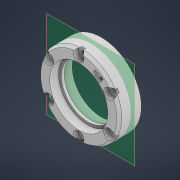
# Autodesk Inventor part: Ring Cover Top
Saved by Autodesk Inventor 2021 (Build 250183000, 183)
## iProperties
Created: 2025-03-19
Part Number: Ring Cover Top
Material: Generic
Document SubType Name: Modeling
Designer: rocke
Density: 0.528258 g/cm^3
Appearance: Default
Mass: 26.1 g
Surface Area: 167.965 cm^2
Volume: 49.4077 cm^3
Author: rocke
Autodesk Inventor part; units mm, degrees
ref_plane "YZ Plane" through (0, 0, 0) normal (1, 0, 0) x (0, 1, 0)
ref_plane "XZ Plane" through (0, 0, 0) normal (0, 1, 0) x (-1, 0, 0)
ref_plane "XY Plane" through (0, 0, 0) normal (0, 0, 1) x (1, 0, 0)
sketch "Sketch1" plane through (0, 0, 0) normal (0, 0, 1) x (1, 0, 0)
  circle A0 centre (0, 0) radius 40
  dimension "d0" = 80
  constraints: 1 centre point, 1 coincident
  measures "d0" diameter of A0
extrude "Extrusion1" add sketch "Sketch1" along normal blind 22.5
sketch "Sketch2" plane through (0, 0, 22.5) normal (0, 0, 1) x (1, 0, 0)
  point P0 (0, 0)
  point P1 (0, 35)
  dimension "d3" = 35
  measures "d3" distance of point (0, 0) point (0, 35)
hole "Hole1" at (0, 35, 22.5) direction (0, 0, -1) diameter 4.3 end through all counterbore diameter 10.59 counterbore depth 5 clearance for "Hex Head Machine Screw" size "M4" standard "Ansi Metric M Profile"
chamfer "Chamfer1" distance 2 distance2 3 2 edges at (-27.6179, -28.9353, 22.5) (28.9353, 27.6179, 22.5) measured on face at (-2.7418, -16.4668, 22.5)
pattern_circular "Circular Pattern1" count 6 over 360 about axis through (0, 0, 0) along (0, 0, 1) of "Hole1"
sketch "Sketch3" plane through (0, 0, 0) normal (0, 0, -1) x (-1, 0, 0)
  circle A0 centre (0, 0) radius 29.1
  dimension "d17" = 58.2
  constraints: 1 centre point, 1 coincident
  measures "d17" diameter of A0
extrude "Extrusion2" cut sketch "Sketch3" against normal through all
ref_plane "Work Plane1" through (0, 0, 10.5) normal (0, 0, -1) x (-1, 0, 0)
sketch "Sketch4" plane through (0, 0, 10.5) normal (0, 0, -1) x (-1, 0, 0)
  circle A0 centre (0, 0) radius 29.5
  circle A1 centre (0, 0) radius 26.5
  dimension "d21" = 53
  dimension "d22" = 59
  constraints: 2 centre point, 2 coincident
  measures "d21" diameter of A1
  measures "d22" diameter of A0
extrude "Extrusion3" add sketch "Sketch4" against normal blind 3
sketch "Sketch5" plane through (0, 0, 22.5) normal (0, 0, 1) x (1, 0, 0)
  arc A0 (33.6722, 21.5913) -> (1.8625, 39.9566) centre (0, 0) ccw projected
  line L0 (0, 0) -> (40, 0) construction
  line L1 (21.3532, 22.5799) -> (24.5138, 27.0811)
  line L2 (24.5138, 27.0811) -> (17.1481, 32.253)
  line L3 (17.1481, 32.253) -> (13.9876, 27.7518)
  line L4 (13.9876, 27.7518) -> (21.3532, 22.5799)
  line L5 (21.3532, 22.5799) -> (17.1481, 32.253) construction
  line L6 (24.5138, 27.0811) -> (13.9876, 27.7518) construction
  line L7 (16.4837, 25.9991) -> (19.6443, 30.5003)
  line L8 (22.0585, 28.8051) -> (18.898, 24.3039)
  line L9 (14.3755, 28.3042) -> (16.7602, 31.7005)
  line L10 (16.7602, 31.7005) -> (19.2564, 29.9479)
  line L11 (19.2564, 29.9479) -> (16.8716, 26.5515)
  line L12 (16.8716, 26.5515) -> (14.3755, 28.3042)
  line L13 (19.2507, 27.4165) -> (15.5679, 30.0024)
  line L14 (16.8716, 26.5515) -> (16.7602, 31.7005)
  line L15 (14.3755, 28.3042) -> (19.2564, 29.9479)
  line L16 (0, 0) -> (16.8159, 29.126)
  line L17 (0, 0) -> (19.2507, 27.4165)
  point P0 (16.8716, 26.5515)
  dimension "d26" = 9
  dimension "d27" = 5.5
  dimension "d29" = 33.5
  dimension "d30" = 3.05
  dimension "d36" = 3
  dimension "d41" = 4.15
  dimension "d42" = 60
  constraints: 36 end point, 6 point on line, 5 parallel, 5 perpendicular, 4 midpoint, 1 collinear, 1 horizontal, 1 other
  measures "d26" distance between parallel lines of L1 L3
  measures "d27" distance between parallel lines of L4 L2
  measures "d29" distance of L16.start L13.start
  measures "d30" distance between parallel lines of L3 L7
  measures "d36" distance between parallel lines of L1 L8
  measures "d41" distance between parallel lines of L12 L10
  measures "d42" angle of L0 L16
extrude "Extrusion4" cut sketch "Sketch5" against normal blind 1.75 contours L4 L17 L13 L7 L2 L8 | L4 L7 L13 L17 | L15 L14 L10 | L7 L13 L15 | L14 L13 L7 | L12 L16 L14 | L14 L13 L3 | L15 L3 L13 | L16 L12 L15
extrude "Extrusion7" cut sketch "Sketch5" against normal through all contours L4 L8 L2 L1
body "Solid1"
